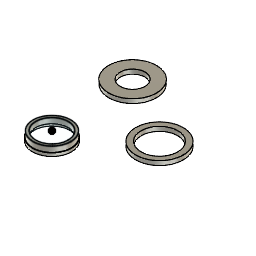
HubCentricRings (Autodesk Fusion 360 design; units mm, degrees)
Autodesk Fusion 360 part; units mm, degrees
sketch "Sketch1" plane through (0, 0, 0) normal (0, 0, 1) x (1, 0, 0)
  line L0 (55, 17.5) -> (82.5, 17.5)
  line L1 (85, 15) -> (85, 10)
  line L2 (82.5, 7.5) -> (55, 7.5)
  arc A0 (85, 15) -> (82.5, 17.5) centre (82.5, 15) ccw
  arc A1 (82.5, 7.5) -> (85, 10) centre (82.5, 10) ccw
  line L3 (55, 17.5) -> (77.9963, 17.5) construction
  line L4 (20.0718, 24.8056) -> (34.9282, 24.8056)
  line L5 (34.9282, 24.8056) -> (55, 17.5)
  line L6 (55, 7.5) -> (34.3939, 0)
  line L7 (55, 7.5) -> (76.9285, 7.5) construction
  line L8 (34.3939, 0) -> (20.6061, 0)
  circle A2 centre (27.5, 12.5) radius 5
  line L9 (34.9282, 24.8056) -> (20.0718, 24.8056)
  line L10 (0, 17.5) -> (-22.9963, 17.5) construction
  line L11 (-30, 15) -> (-30, 10)
  arc A3 (-30, 10) -> (-27.5, 7.5) centre (-27.5, 10) ccw
  line L12 (0, 7.5) -> (-21.9285, 7.5) construction
  line L13 (0, 7.5) -> (20.6061, 0)
  line L14 (0, 17.5) -> (-27.5, 17.5)
  line L15 (20.0718, 24.8056) -> (0, 17.5)
  arc A4 (-27.5, 17.5) -> (-30, 15) centre (-27.5, 15) ccw
  line L16 (-27.5, 7.5) -> (0, 7.5)
  line L17 (20.6061, 0) -> (34.3939, 0)
  circle A5 centre (27.5, 12.5) radius 5
  point P0 (85, 17.5)
  point P1 (27.5, -12)
  point P2 (27.5, 34)
  point P3 (-30, 17.5)
  dimension "d5" = 30
  dimension "d6" = 10
  dimension "d16" = 160
  dimension "d17" = 10
  constraint horizontal L0
  constraint vertical L1
  constraint horizontal L2
  constraint coincident P0 L0
  constraint coincident P0 L1
  constraint tangent L0 A0
  constraint tangent L1 A0
  constraint tangent L1 A1
  constraint tangent L2 A1
  constraint horizontal L3
  constraint horizontal L4
  constraint horizontal L7
  constraint horizontal L8
  measures "d5" distance of L0.start P0
  measures "d6" distance of L0.start L2.end
  measures "d16" angle of L6 L7
  measures "d17" diameter of A2
sketch "Sketch2" plane through (0, 0, 0) normal (0, 0, 1) x (1, 0, 0)
  circle A0 centre (0, 0) radius 35
  circle A1 centre (0, 0) radius 30
  dimension "d18" = 70
  dimension "d19" = 60
  constraint coincident A0.centre A1.centre
  measures "d18" diameter of A0
  measures "d19" diameter of A1
extrude "Extrude2" add sketch "Sketch2" against normal blind 10 draft 2 contours A0 | A1 makes body 1
extrude "Extrude3" cut sketch "Sketch2" against normal blind 20 contours A1 bodies 1
sketch "Sketch3" plane through (0, 0, -10) normal (0, 0, -1) x (1, 0, 0)
  circle A0 centre (0, 0) radius 30
  circle A1 centre (0, 0) radius 35.3492
  circle A2 centre (0, 0) radius 36.3492
  circle A3 centre (0, 0) radius 33
  dimension "d29" = 1
  dimension "d30" = 3
extrude "Extrude4" add sketch "Sketch3" along normal blind 6 contours A1 | A2 bodies 1
sketch "Sketch4" plane through (0, 0, 0) normal (0, 0, 1) x (1, 0, 0)
  circle A0 centre (0, 150) radius 44.25
  dimension "d33" = 88.5
  measures "d33" diameter of A0
extrude "Extrude5" add sketch "Sketch4" along normal blind 8 draft 2 separate body makes body 2
sketch "Sketch5" plane through (0, 0, 8) normal (0, 0, 1) x (-1, 0, 0)
  circle A0 centre (0, -150) radius 44.5294
  circle A1 centre (0, -150) radius 23
  dimension "d36" = 46
  constraint concentric A0 A1
  measures "d36" diameter of A1
extrude "Extrude6" cut sketch "Sketch5" against normal blind 8 draft -2 contours A1 bodies 2
sketch "Sketch6" plane through (0, 0, 0) normal (0, 0, 1) x (1, 0, 0)
  circle A0 centre (125, 75) radius 44.25
  dimension "d39" = 88.5
  measures "d39" diameter of A0
extrude "Extrude7" add sketch "Sketch6" along normal blind 8 separate body makes body 3
sketch "Sketch7" plane through (0, 0, 8) normal (0, 0, 1) x (-1, 0, 0)
  circle A0 centre (-125, -75) radius 44.25
  circle A1 centre (-125, -75) radius 34
  dimension "d42" = 68
  constraint concentric A0 A1
  measures "d42" diameter of A1
extrude "Extrude8" cut sketch "Sketch7" against normal blind 8 draft -2 contours A1 bodies 3
sketch "Sketch8" plane through (0, 0, 0) normal (0, 0, -1) x (1, 0, 0)
  circle A0 centre (0, -150) radius 22.7206
  circle A1 centre (0, -150) radius 44.25
  line L0 (-10, -125) -> (10, -125) construction
  line L1 (10, -125) -> (10, -115) construction
  line L2 (10, -115) -> (-10, -115) construction
  line L3 (-10, -115) -> (-10, -125) construction
  line L4 (115, -40) -> (135, -40) construction
  line L5 (135, -40) -> (135, -35) construction
  line L6 (135, -35) -> (115, -35) construction
  line L7 (115, -35) -> (115, -40) construction
  dimension "d45" = 7
  dimension "d46" = 5
  text T0 "OUT" font "Arial" height 7 align left top in box 20 x 10 at (-10, -125) x (1, 0) y (0, 1) spacing 1
  text T1 "OUT" font "Arial" height 5 align left top in box 20 x 5 at (115, -40) x (1, 0) y (0, 1) spacing 1
extrude "Extrude9" cut sketch "Sketch8" against normal blind 1 text T1 T0 bodies 2 3
named bodies: "Rear Hubcentric", "Front Hubcentric"
